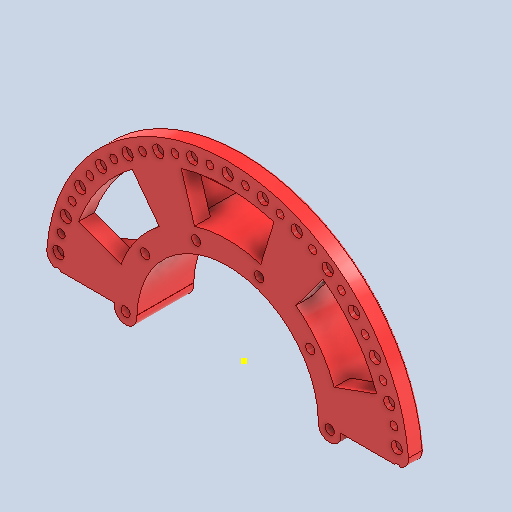
# Autodesk Inventor part: モーターマウント板固定部品
Saved by Autodesk Inventor 2024 (Build 280153000, 153)
## iProperties
Created: 2023-05-30
Part Number: モーターマウント板固定部品
Material: 一般
Document SubType Name: Modeling
Designer: yuta2
Density: 1 g/cm^3
Appearance: 淡い赤
Mass: 64.5602 g
Surface Area: 263.323 cm^2
Volume: 64.5602 cm^3
Author: yuta2
Autodesk Inventor part; units mm, degrees
ref_plane "YZ Plane" through (0, 0, 0) normal (1, 0, 0) x (0, 1, 0)
ref_plane "XZ Plane" through (0, 0, 0) normal (0, 1, 0) x (-1, 0, 0)
ref_plane "XY Plane" through (0, 0, 0) normal (0, 0, 1) x (1, 0, 0)
sketch "スケッチ1" plane through (0, 0, 0) normal (0, 0, 1) x (1, 0, 0)
  circle A0 centre (0, 0) radius 80
  circle A1 centre (0, 0) radius 70
  circle A2 centre (0, 0) radius 40
  circle A3 centre (0, 0) radius 50
  circle A4 centre (45, 0) radius 5
  circle A5 centre (-45, 0) radius 5
  line L0 (79.9937, 1) -> (-79.9937, 1)
  line L1 (0, 0) -> (65.7785, 23.9414)
  line L2 (0, 0) -> (42.1271, 55.9045)
  line L3 (0, 0) -> (0.7536, 1)
  line L4 (20.466, 66.9413) -> (0, 0)
  line L5 (0, 0) -> (0, 40)
  line L6 (0, 0) -> (-65.7785, 23.9414)
  line L7 (0, 0) -> (-42.1271, 55.9045)
  line L8 (-20.466, 66.9413) -> (0, 0)
  point P0 (75.1754, 27.3616)
  point P1 (48.1452, 63.8908)
  point P2 (23.3897, 76.5044)
  point P3 (-75.1754, 27.3616)
  point P4 (-48.1452, 63.8908)
  point P5 (-23.3897, 76.5044)
  point P6 (46.9846, 17.101)
  point P7 (30.0908, 39.9318)
  point P8 (-30.0908, 39.9318)
  point P9 (-46.9846, 17.101)
  point P10 (-49.899, 1)
  point P11 (-40.101, 1)
  point P12 (-39.9875, 1)
  point P13 (39.9875, 1)
  point P14 (40.101, 1)
  point P15 (49.899, 1)
  point P16 (14.6186, 47.8152)
  point P17 (-14.6186, 47.8152)
  dimension "d2" = 80
  dimension "d0" = 160
  dimension "d1" = 10
  dimension "d3" = 100
  dimension "d4" = 1
  dimension "d5" = 20
  dimension "d6" = 20
  dimension "d7" = 33
  constraints: 18 end point, 11 point on circle, 5 centre point, 3 coincident, 3 symmetric about line, 2 horizontal alignment, 2 point on line, 2 tangent, 1 horizontal, 1 vertical, 8 other
  measures "d0" diameter of A0
  measures "d1" radial gap between concentric circles of A0 A1
  measures "d3" diameter of A3
  measures "d4" distance from line of point (0, 0) L0
  measures "d5" angle of L0 L1
  measures "d6" angle of L4 L2
  measures "d7" angle of L1 L2
extrude "押し出し1" add sketch "スケッチ1" along normal blind 7 contours L0 A1 A0 | L0 A3 L1 A1 | A1 L6 A3 L0 | L0 A4 A2 L1 A3 | A3 L6 A2 L0 A5 | L2 A3 L4 A1 | L1 A2 L2 A3 | A4 L0 | L0 A4 | A1 L8 A3 L7 | A3 L7 A2 L6 | A5 L0 | A5 L0 | L2 A2 L4 A3 | A3 L8 A2 L7 | L4 A2 L8 A3 picked at (-7.5875, 76.0873)
sketch "スケッチ2" plane through (0, 0, 7) normal (0, 0, 1) x (1, 0, 0)
  circle A0 centre (0, 0) radius 75
  line L0 (74.5891, 7.8396) -> (0, 0)
  line L1 (0, 0) -> (75, 0)
  dimension "d10" = 150
  dimension "d11" = 6
  constraints: 4 end point, 2 point on circle, 1 centre point, 1 coincident, 1 horizontal
  measures "d10" diameter of A0
  measures "d11" angle of L1 L0
hole "穴1" at (74.5891, 7.8396, 7) direction (0, 0, -1) diameter 5 depth 2
pattern_circular "円形状パターン1" count 15 over 168 about axis through (0, 0, 0) along (0, 0, 1) of "穴1"
sketch "スケッチ3" plane through (0, 0, 0) normal (0, 0, -1) x (-1, 0, 0)
  arc A0 (79.9937, 1) -> (-79.9937, 1) centre (0, 0) ccw projected
  line L0 (-49.899, 1) -> (-79.9937, 1) projected
  arc A1 (-49.899, 1) -> (-40.101, 1) centre (-45, 0) ccw projected
  line L1 (-39.9875, 1) -> (-40.101, 1) projected
  arc A2 (39.9875, 1) -> (-39.9875, 1) centre (0, 0) ccw projected
  line L2 (40.101, 1) -> (39.9875, 1) projected
  arc A3 (40.101, 1) -> (49.899, 1) centre (45, 0) ccw projected
  line L3 (79.9937, 1) -> (49.899, 1) projected
  arc A4 (-42.1271, 55.9045) -> (-65.7785, 23.9414) centre (0, 0) ccw projected
  line L4 (-30.0908, 39.9318) -> (-42.1271, 55.9045) projected
  arc A5 (-30.0908, 39.9318) -> (-46.9846, 17.101) centre (0, 0) ccw projected
  line L5 (-65.7785, 23.9414) -> (-46.9846, 17.101) projected
  arc A6 (65.7785, 23.9414) -> (42.1271, 55.9045) centre (0, 0) ccw projected
  line L6 (46.9846, 17.101) -> (65.7785, 23.9414) projected
  arc A7 (46.9846, 17.101) -> (30.0908, 39.9318) centre (0, 0) ccw projected
  line L7 (42.1271, 55.9045) -> (30.0908, 39.9318) projected
  line L8 (-20.466, 66.9413) -> (-14.6186, 47.8152) projected
  arc A8 (20.466, 66.9413) -> (-20.466, 66.9413) centre (0, 0) ccw projected
  line L9 (14.6186, 47.8152) -> (20.466, 66.9413) projected
  arc A9 (14.6186, 47.8152) -> (-14.6186, 47.8152) centre (0, 0) ccw projected
  circle A10 centre (0, 0) radius 50
  circle A11 centre (0, 0) radius 45
  line L10 (45, 0) -> (0, 0)
  line L11 (0, 0) -> (45, 0)
  point P0 (49.99, 1)
  point P1 (30.0908, 39.9318)
  point P2 (-49.99, 1)
  dimension "d32" = 90
  dimension "d33" = 0
  constraints: 4 end point, 3 coincident, 1 horizontal, 1 horizontal alignment, 5 other
  measures "d33" distance between parallel lines of L11 L10
extrude "押し出し2" add sketch "スケッチ3" along normal blind 18 contours L3 A3 A11 A1 L0 A10 A5 A9 A7 | A3 L10 A11 | A11 L10 A3 L2 A2 L1 A1
sketch "スケッチ4" plane through (0, 0, 0) normal (0, 0, -1) x (-1, 0, 0)
  arc A0 (-46.9846, 17.101) -> (-49.99, 1) centre (0, 0) ccw projected
  line L0 (-49.6129, 6.2095) -> (-48.7447, 11.1336)
  line L1 (-48.7447, 11.1336) -> (-68.4584, 14.6096)
  line L2 (-68.4584, 14.6096) -> (-69.3267, 9.6856)
  line L3 (-69.3267, 9.6856) -> (-49.6129, 6.2095)
  arc A1 (30.0908, 39.9318) -> (14.6186, 47.8152) centre (0, 0) ccw projected
  line L4 (42.1271, 55.9045) -> (30.0908, 39.9318) projected
  arc A2 (65.7785, 23.9414) -> (42.1271, 55.9045) centre (0, 0) ccw projected
  line L5 (46.9846, 17.101) -> (65.7785, 23.9414) projected
  arc A3 (49.99, 1) -> (46.9846, 17.101) centre (0, 0) ccw projected
  line L6 (79.9937, 1) -> (49.99, 1) projected
  arc A4 (79.9937, 1) -> (-79.9937, 1) centre (0, 0) ccw projected
  line L7 (-49.99, 1) -> (-79.9937, 1) projected
  arc A5 (-46.9846, 17.101) -> (-49.99, 1) centre (0, 0) ccw projected
  line L8 (-65.7785, 23.9414) -> (-46.9846, 17.101) projected
  arc A6 (-42.1271, 55.9045) -> (-65.7785, 23.9414) centre (0, 0) ccw projected
  line L9 (-30.0908, 39.9318) -> (-42.1271, 55.9045) projected
  arc A7 (-14.6186, 47.8152) -> (-30.0908, 39.9318) centre (0, 0) ccw projected
  line L10 (-20.466, 66.9413) -> (-14.6186, 47.8152) projected
  arc A8 (20.466, 66.9413) -> (-20.466, 66.9413) centre (0, 0) ccw projected
  line L11 (14.6186, 47.8152) -> (20.466, 66.9413) projected
  circle A9 centre (0, 0) radius 70
  line L12 (-49.99, 1) -> (-79.9937, 1) projected
  arc A10 (49.99, 1) -> (-49.99, 1) centre (0, 0) ccw projected
  line L13 (-20.4436, 45.6296) -> (-24.8986, 43.3596)
  line L14 (-24.8986, 43.3596) -> (-33.9862, 61.1949)
  line L15 (-33.9862, 61.1949) -> (-29.5311, 63.4649)
  line L16 (-29.5311, 63.4649) -> (-20.4436, 45.6296)
  line L17 (-30.0908, 39.9318) -> (-42.1271, 55.9045) projected
  line L18 (0, 0) -> (0, 50)
  line L19 (48.7447, 11.1336) -> (68.4584, 14.6096)
  line L20 (69.3267, 9.6856) -> (49.6129, 6.2095)
  line L21 (24.8986, 43.3596) -> (33.9862, 61.1949)
  line L22 (29.5311, 63.4649) -> (20.4436, 45.6296)
  line L23 (33.9866, 61.1957) -> (24.8986, 43.3596)
  line L24 (29.5311, 63.4649) -> (20.4436, 45.6296)
  line L25 (-33.9862, 61.1949) -> (-24.8986, 43.3596)
  line L26 (-20.4436, 45.6296) -> (-29.5311, 63.4649)
  line L27 (29.5315, 63.4656) -> (20.4436, 45.6296)
  dimension "d25" = 5
  dimension "d26" = 10
  dimension "d27" = 10
  dimension "d28" = 5
  constraints: 36 end point, 8 symmetric about line, 7 point on circle, 6 parallel, 2 collinear, 2 perpendicular, 1 centre point, 1 coincident, 1 point on line, 4 other
  measures "d25" distance between parallel lines of L1 L3
  measures "d26" angle of L12 L3
  measures "d27" angle of L17 L14
  measures "d28" distance between parallel lines of L14 L16
extrude "押し出し3" add sketch "スケッチ4" along normal blind 20 contours A0 L3 L2 L1 | L14 L15 L16 A7 | L20 A3 L19 A9 | A9 L21 A1 L22
sketch "スケッチ5" plane through (49.6129, 6.2095, -20) normal (0.1736482, -0.9848078, 0) x (0.9848078, 0.1736482, 0)
  line L0 (0, 20) -> (20.0179, 20) projected
  line L1 (0, 2) -> (0, 20) projected
  line L2 (20.0179, 0) -> (0, 0) projected
  line L3 (20.0179, 20) -> (20.0179, 0) projected
  line L4 (20.0179, 20) -> (0, 0)
  line L5 (-49.9375, 20) -> (-49.9375, -35.5638)
  line L6 (20.0179, 0) -> (29.0147, 0)
  line L7 (29.0147, 0) -> (29.0147, 20)
  line L8 (29.0147, 20) -> (20.0179, 20)
  line L9 (20.0179, 20) -> (20.0179, 0)
  line L10 (0, 2) -> (0, 0) projected
  line L11 (-17.8878, 2) -> (0, 2) projected
  line L12 (-17.8878, 2) -> (29.0147, 2)
  point P0 (2.0018, 2)
  point P1 (0, 2)
  constraints: 14 end point, 2 parallel, 2 perpendicular, 1 horizontal, 1 point on line, 1 vertical
revolve "回転1" cut sketch "スケッチ5" angle 360 about axis through (0.4341, -2.462, 0) along (0, 0, -1) contours L8 L7 L12 L3 | L3 L12 L4 | L12 L4 L10 | L12 L7 L6 L3 | L3 L2 L4 L12
sketch "スケッチ6" plane through (0, 0, -18) normal (0, 0, -1) x (-1, 0, 0)
  arc A0 (40.101, 1) -> (49.899, 1) centre (45, 0) ccw projected
  point P0 (0, 0)
  constraints: 1 coincident
hole "穴2" at (-45, 0, -18) direction (0, 0, 1) diameter 4.1 end through all counterbore diameter 5.8 counterbore depth 4
pattern_circular "円形状パターン2" count 6 over 180 about axis through (0, 0, 0) along (0, 0, -1) of "穴2"
fillet "フィレット1" radius 5 2 edges at (-79.9937, 1, 3.5) (79.9937, 1, 3.5)
fillet "フィレット2" radius 1 9 edges at (60.1469, 1, 0) (72.5317, 1, 0) (77.3148, 1.7022, 0) (79.6508, 4.9628, 0) (0, 80, 0) (-79.4677, 4.3165, 0) (-76.7157, 1.3985, 0) (-72.0976, 1, 0) (-59.7128, 1, 0)
sketch "スケッチ7" plane through (0, 0, 0) normal (0, 0, -1) x (-1, 0, 0)
  circle A0 centre (0, 0) radius 75
  line L0 (-7.8396, 74.5891) -> (0, 0)
  line L1 (0, 0) -> (0, 40)
  arc A1 (39.9875, 1) -> (-39.9875, 1) centre (0, 0) ccw projected
  dimension "d46" = 150
  dimension "d57" = 6
  constraints: 4 end point, 1 coincident, 1 point on circle, 1 vertical, 3 other
  measures "d57" angle of L1 L0
hole "穴3" at (7.8396, 74.5891, 0) direction (0, 0, 1) diameter 3.5 end through all
pattern_circular "円形状パターン3" count 30 over 360 about axis through (0, 0, 0) along (0, 0, 1) of "穴3"
sketch "スケッチ8" plane through (0, 0, 0) normal (0, 0, -1) x (-1, 0, 0)
  point P0 (0, 0)
equation "\"d10\" = D"
equation "\"d46\" = D"
equation "\"D\" = 150"
